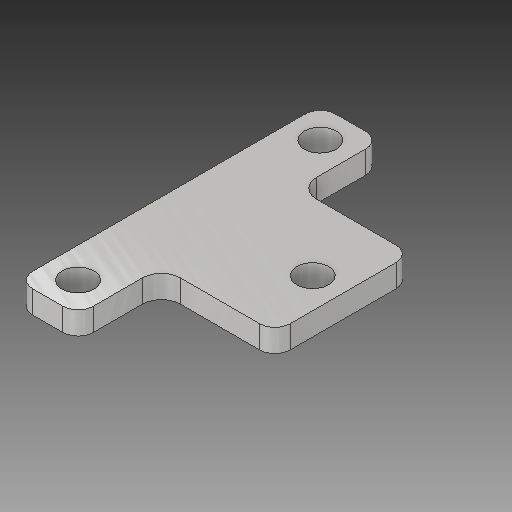
# Autodesk Inventor part: T_almite_braket
Saved by Autodesk Inventor 2018 (Build 220112000, 112)
## iProperties
Created: 2020-07-22
Part Number: T_almite_braket
Material: 一般
Document SubType Name: Sheet Metal
Designer: gisen
Density: 1 g/cm^3
Sheet Metal Rule: Default_mm
Appearance: 機械加工 - アルミニウム
Mass: 1.63791 g
Surface Area: 15.668 cm^2
Volume: 1.63791 cm^3
Author: gisen
Autodesk Inventor part; units mm, degrees
ref_plane "YZ Plane" through (0, 0, 0) normal (1, 0, 0) x (0, 1, 0)
ref_plane "XZ Plane" through (0, 0, 0) normal (0, 1, 0) x (-1, 0, 0)
ref_plane "XY Plane" through (0, 0, 0) normal (0, 0, 1) x (1, 0, 0)
sketch "スケッチ1" plane through (0, 0, 0) normal (0, 1, 0) x (-1, 0, 0)
  line L0 (-3, 9) -> (10, 9)
  line L1 (10, -9) -> (-3, -9)
  line L2 (-5, -7) -> (-5, 7)
  line L3 (12, 20) -> (16, 20)
  line L4 (18, 18) -> (18, -18)
  line L5 (16, -20) -> (12, -20)
  line L6 (10, -18) -> (10, -9)
  line L7 (10, 9) -> (10, 18)
  arc A0 (18, 18) -> (16, 20) centre (16, 18) ccw
  arc A1 (12, 20) -> (10, 18) centre (12, 18) ccw
  arc A2 (16, -20) -> (18, -18) centre (16, -18) ccw
  arc A3 (10, -18) -> (12, -20) centre (12, -18) ccw
  arc A4 (-5, -7) -> (-3, -9) centre (-3, -7) ccw
  arc A5 (-3, 9) -> (-5, 7) centre (-3, 7) ccw
  point P0 (0, 0)
  point P1 (-5, 9)
  point P2 (-5, -9)
  point P3 (10, 20)
  point P4 (18, -20)
  point P5 (18, 20)
  point P6 (10, -20)
  dimension "d0" = 5
  dimension "d2" = 8
  dimension "d3" = 8
  dimension "d4" = 18
  dimension "d5" = 9
  dimension "d6" = 40
  dimension "d7" = 20
  dimension "d8" = 10
  dimension "d10" = 2
  measures "d0" distance from line of L2 point (0, 0)
  measures "d2" distance between parallel lines of L6 L4
  measures "d3" distance between parallel lines of L7 L4
  measures "d4" distance between parallel lines of L0 L1
  measures "d5" distance from line of L0 point (0, 0)
  measures "d6" distance between parallel lines of L5 L3
  measures "d7" distance from line of point (0, 0) L5
  measures "d8" distance from line of point (0, 0) L6
  measures "d10" radius of A0
extrude "プレート1" add sketch "スケッチ1" along normal blind 3
hole "穴1" at (-14, 3, 16) direction (0, -1, 0) diameter 4.2 end through all
hole "穴2" at (-14, 3, -16) direction (0, -1, 0) diameter 4.2 end through all
hole "穴3" at (1, 3, 0) direction (0, -1, 0) diameter 4.2 end through all
sketch "スケッチ2" plane through (0, 0, 0) normal (0, -1, 0) x (1, 0, 0)
  circle A0 centre (1, 0) radius 2.1 projected
  circle A1 centre (-14, -16) radius 2.1 projected
  circle A2 centre (-14, 16) radius 2.1 projected
  line L0 (-10, 9) -> (3, 9) projected
  line L1 (-10, 18) -> (-10, 9) projected
  arc A3 (-10, 18) -> (-12, 20) centre (-12, 18) ccw projected
  line L2 (-16, 20) -> (-12, 20) projected
  arc A4 (-16, 20) -> (-18, 18) centre (-16, 18) ccw projected
  line L3 (-18, -18) -> (-18, 18) projected
  arc A5 (-18, -18) -> (-16, -20) centre (-16, -18) ccw projected
  line L4 (-12, -20) -> (-16, -20) projected
  arc A6 (-12, -20) -> (-10, -18) centre (-12, -18) ccw projected
  line L5 (-10, -9) -> (-10, -18) projected
  line L6 (3, -9) -> (-10, -9) projected
  arc A7 (3, -9) -> (5, -7) centre (3, -7) ccw projected
  line L7 (5, 7) -> (5, -7) projected
  arc A8 (5, 7) -> (3, 9) centre (3, 7) ccw projected
  point P0 (0, 0)
fillet "フィレット1" radius 2.5 2 edges at (-10, 1.5, 9) (-10, 1.5, -9)
equation "\"d3\" = d2"
equation "\"d18\" = Thickness"
equation "\"d28\" = Thickness"
equation "\"d37\" = Thickness"
equation "\"d9\" = Thickness"
equation "\"d5\" = 0.5 * d4"
equation "\"d7\" = 0.5 * d6"
equation "\"BendRadius\" = Thickness"
equation "\"BendReliefWidth\" = Thickness"
equation "\"BendReliefDepth\" = 0.5 * Thickness"
equation "\"CornerReliefSize\" = 4 * Thickness"
equation "\"MinimumRemnant\" = 2 * Thickness"
equation "\"TransitionRadius\" = BendRadius"
equation "\"JacobiRadiusSize\" = BendRadius"
equation "\"GapSize\" = Thickness"
equation "\"Thickness\" = 3"
